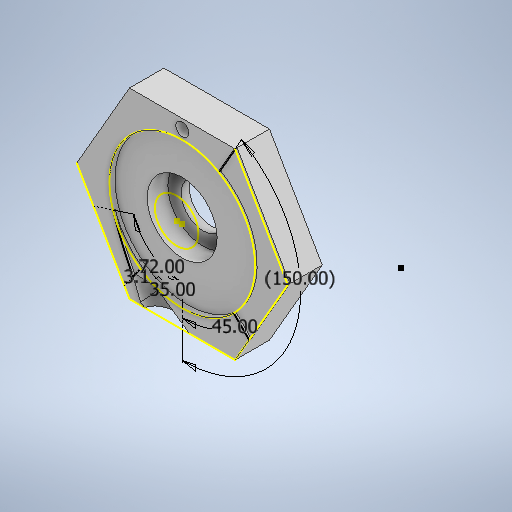
# Autodesk Inventor part: Case
Saved by Autodesk Inventor 2026.1 (Build 301233020, 233B)
## iProperties
Created: 2025-10-20
Part Number: Case
Material: Generic
Document SubType Name: Modeling
Designer: yo
Density: 1 g/cm^3
Appearance: Default
Author: yo
Autodesk Inventor part; units mm, degrees
ref_plane "YZ Plane" through (0, 0, 0) normal (1, 0, 0) x (0, 1, 0)
ref_plane "XZ Plane" through (0, 0, 0) normal (0, 1, 0) x (-1, 0, 0)
ref_plane "XY Plane" through (0, 0, 0) normal (0, 0, 1) x (1, 0, 0)
sketch "Sketch1" plane through (0, 0, 0) normal (0, 0, 1) x (1, 0, 0)
  circle A0 centre (0, 0) radius 17.6
  line L0 (-12.7594, 22.1) -> (12.7594, 22.1)
  line L1 (12.7594, 22.1) -> (25.5189, 0)
  line L2 (25.5189, 0) -> (12.7594, -22.1)
  line L3 (12.7594, -22.1) -> (-12.7594, -22.1)
  line L4 (-12.7594, -22.1) -> (-25.5189, 0)
  line L5 (-25.5189, 0) -> (-12.7594, 22.1)
  circle A1 centre (0, 19.85) radius 1.55
  line L6 (0, 22.1) -> (0, 17.6) construction
  circle A2 centre (-1.35, 0) radius 5.25
  circle A3 centre (-1.35, 0) radius 8.45
  point P0 (-17.6, 0)
  dimension "d0" = 35.2
  dimension "d1" = 3.1
  dimension "d2" = 4.5
  dimension "d23" = 10.5
  dimension "d24" = 16.9
  dimension "d25" = 16.25
  constraints: 14 end point, 4 centre point, 4 coincident, 2 horizontal alignment, 2 midpoint, 2 point on circle, 1 horizontal, 1 vertical, 13 other
  measures "d0" diameter of A0
  measures "d1" diameter of A1
  measures "d2" distance of L6.start L6.end
  measures "d23" diameter of A2
  measures "d24" diameter of A3
  measures "d25" distance of A2.centre A0.end
extrude "Extrusion1" add sketch "Sketch1" along normal blind 2 contours A3
extrude "Extrusion2" add sketch "Sketch1" along normal blind 7 contours A0
extrude "Extrusion3" add sketch "Sketch1" along normal blind 8.325 contours L0 L1 L2 L3 L4 L5
sketch "Sketch2" plane through (0, 0, 8.325) normal (0, 0, 1) x (1, 0, 0)
  circle A0 centre (0, 0) radius 17.6 projected
  line L0 (0, -17.6) -> (0, -22.1) construction
  line L1 (-12.7594, -22.1) -> (12.7594, -22.1) projected
  line L2 (-10.0949, -14.4171) -> (-13.9865, -19.9747) construction
  line L3 (-16.7386, -5.4387) -> (-21.4879, -6.9818) construction
  line L4 (8.8, 15.242) -> (12.7594, 22.1)
  line L5 (12.4451, -12.4451) -> (16.1783, -16.1783)
  line L6 (12.7594, -22.1) -> (25.5189, 0) projected
  line L7 (25.5189, 0) -> (12.7594, 22.1) projected
  line L8 (-25.5189, 0) -> (-12.7594, -22.1) projected
  circle A1 centre (-1.35, 0) radius 5.25 projected
  line L9 (-10.0949, -14.4171) -> (-11.873, -16.9564)
  arc A2 (-16.7386, -5.4387) -> (-11.873, -16.9564) centre (52.8526, 17.1728) ccw
  dimension "d15" = 35
  dimension "d16" = 72
  dimension "d18" = 150
  dimension "d19" = 45
  dimension "d45" = 3.1
  constraints: 12 end point, 7 point on circle, 4 line through centre, 4 point on line, 1 centre point, 1 midpoint, 1 tangent, 1 vertical
  measures "d15" angle of L0 L2
  measures "d16" angle of L0 L3
  measures "d18" angle of L4 L0
  measures "d19" angle of L0 L5
  measures "d45" distance of L9.end L2.start
extrude "Extrusion4" cut sketch "Sketch2" against normal blind 0.5 contours A0 L4 L7 L6 L5
extrude "Extrusion5" cut sketch "Sketch2" against normal blind 0.5 contours A0 L9 A2
ref_plane "Work Plane1" through (0, 0, 8.325) normal (0, 0, 1) x (1, 0, 0)
sketch "Sketch3" plane through (0, 0, 8.325) normal (0, 0, 1) x (1, 0, 0)
  line L0 (-10.0949, -14.4171) -> (-11.873, -16.9564) projected
  line L1 (-10.984, -15.6868) -> (-10.0949, -14.4171)
  line L2 (-11.5862, -16.5469) -> (8.0734, -30.3127)
  line L3 (-10.0877, -21.3805) -> (6.2953, -32.8521)
  line L4 (-10.0877, -21.3805) -> (-11.873, -16.9564)
  line L5 (6.2953, -32.8521) -> (8.0734, -30.3127)
  point P0 (0, 0)
  dimension "d36" = 6.2
  dimension "d39" = 4
  dimension "d41" = 20
  dimension "d43" = 1
  constraints: 10 end point, 2 perpendicular, 1 collinear, 1 midpoint, 1 parallel, 1 point on line
  measures "d36" diameter of L3 L2
  measures "d39" distance from line of L3.start L0
  measures "d41" distance of L3.start L3.end
  measures "d43" diameter of L0.end L2
revolve "Revolution1" cut sketch "Sketch3" angle 360 about axis through (-11.5862, -16.5469, 8.325) along (0.819152, -0.5735764, 0)
body "Solid1"
